Autodesk Inventor part; units mm, degrees
(part 2 of 2)
sketch "Magnet_flange_bottom_front" plane through (0, 0, -10) normal (0, 0, -1) x (-1, 0, 0)
  circle A0 centre (-365, 62.5) radius 1.65
  arc A1 (-385, 56.5) -> (-385, 68.5) centre (-385, 62.5) ccw
  line L0 (-355, 52.5) -> (-355, 72.5)
  line L1 (-355, 52.5) -> (-370, 52.5)
  circle A2 centre (-377.5, 45) radius 2.25
  line L2 (-370, 52.5) -> (-370, 37.5)
  line L3 (-385, 56.5) -> (-385, 37.5)
  line L4 (-385, 37.5) -> (-370, 37.5)
  line L5 (-385, 87.5) -> (-385, 68.5)
  line L6 (-370, 87.5) -> (-385, 87.5)
  line L7 (-370, 72.5) -> (-370, 87.5)
  line L8 (-355, 72.5) -> (-370, 72.5)
  circle A3 centre (-377.5, 80) radius 2.25
  point P0 (0, 0)
  dimension "d739" = 50
  dimension "d740" = 15
  dimension "d741" = 15
  dimension "d742" = 15
  dimension "d743" = 4.5
  dimension "d744" = 4.5
  dimension "d745" = 7.5
  dimension "d746" = 7.5
  dimension "d747" = 12
  dimension "d748" = 15
  dimension "d749" = 15
  dimension "d750" = 7.5
  dimension "d751" = 7.5
  dimension "d752" = 19
  dimension "d753" = 3.3
  dimension "d754" = 10
  dimension "d755" = 10
  constraints: 18 end point, 4 centre point, 3 parallel, 3 perpendicular, 2 line through centre, 2 point on circle, 1 coincident
  measures "d739" distance between parallel lines of L6 L4
  measures "d740" distance between parallel lines of L4 L1
  measures "d741" distance between parallel lines of L6 L8
  measures "d742" distance between parallel lines of L0 L2
  measures "d743" diameter of A2
  measures "d744" diameter of A3
  measures "d745" distance from line of L4 A2.centre
  measures "d746" distance from line of L6 A3.centre
  measures "d747" diameter of A1
  measures "d748" distance between parallel lines of L3 L2
  measures "d749" distance between parallel lines of L5 L7
  measures "d750" distance from line of L2 A2.centre
  measures "d751" distance from line of L7 A3.centre
  measures "d752" distance of L3.start L4.start
  measures "d753" diameter of A0
  measures "d754" distance from line of L1 A0.centre
  measures "d755" distance from line of L0 A0.centre
sketch "Magnet_flange_middle_front" plane through (0, 0, -10) normal (0, 0, -1) x (-1, 0, 0)
  circle A0 centre (-415, 355) radius 1.65
  arc A1 (-435, 349) -> (-435, 361) centre (-435, 355) ccw
  line L0 (-405, 345) -> (-405, 365)
  line L1 (-405, 345) -> (-420, 345)
  circle A2 centre (-427.5, 337.5) radius 2.25
  line L2 (-420, 345) -> (-420, 330)
  line L3 (-435, 349) -> (-435, 330)
  line L4 (-435, 330) -> (-420, 330)
  line L5 (-435, 380) -> (-435, 361)
  line L6 (-420, 380) -> (-435, 380)
  line L7 (-420, 365) -> (-420, 380)
  line L8 (-405, 365) -> (-420, 365)
  circle A3 centre (-427.5, 372.5) radius 2.25
  point P0 (0, 0)
  dimension "d756" = 50
  dimension "d757" = 15
  dimension "d758" = 15
  dimension "d759" = 15
  dimension "d760" = 4.5
  dimension "d761" = 4.5
  dimension "d762" = 7.5
  dimension "d763" = 7.5
  dimension "d764" = 12
  dimension "d765" = 15
  dimension "d766" = 15
  dimension "d767" = 7.5
  dimension "d768" = 7.5
  dimension "d769" = 19
  dimension "d770" = 3.3
  dimension "d771" = 10
  dimension "d772" = 10
  constraints: 18 end point, 4 centre point, 3 parallel, 3 perpendicular, 2 line through centre, 2 point on circle, 1 coincident
  measures "d756" distance between parallel lines of L6 L4
  measures "d757" distance between parallel lines of L4 L1
  measures "d758" distance between parallel lines of L6 L8
  measures "d759" distance between parallel lines of L0 L2
  measures "d760" diameter of A2
  measures "d761" diameter of A3
  measures "d762" distance from line of L4 A2.centre
  measures "d763" distance from line of L6 A3.centre
  measures "d764" diameter of A1
  measures "d765" distance between parallel lines of L3 L2
  measures "d766" distance between parallel lines of L5 L7
  measures "d767" distance from line of L2 A2.centre
  measures "d768" distance from line of L7 A3.centre
  measures "d769" distance of L3.start L3.end
  measures "d770" diameter of A0
  measures "d771" distance from line of L1 A0.centre
  measures "d772" distance from line of L0 A0.centre
extrude "Magnet_flange_middle_front_1" add sketch "Magnet_flange_middle_front" along normal blind 10 separate body
extrude "Magnet_flange_bottom_front_1" add sketch "Magnet_flange_bottom_front" along normal blind 10 separate body
sketch "Magnet_hole_top_door_front" plane through (0, 0, 10) normal (0, 0, 1) x (1, 0, 0)
  line L0 (185, 580) -> (375, 580) projected
  line L1 (380, 575) -> (380, 485) projected
  point P0 (0, 0)
  point P1 (390, 530)
  dimension "d811" = 50
  dimension "d812" = 10
  measures "d811" distance from line of point (390, 530) L0
  measures "d812" distance from line of L1 point (390, 530)
hole "Magnet_hole_top_door_front_1" at (390, 530, 10) direction (0, 0, -1) diameter 6.2 end through all bodies 1
sketch "Top_door_hinge_levellers_front_holes" plane through (0, 0, 10) normal (0, 0, 1) x (1, 0, 0)
  line L0 (565, 610) -> (0, 610) projected
  line L1 (0, 610) -> (0, 0) projected
  point P0 (147.3, 580.9)
  point P1 (147.3, 549.1)
  point P2 (147.3, 510.9)
  point P3 (147.3, 479.1)
  dimension "d850" = 29.1
  dimension "d851" = 147.3
  dimension "d852" = 31.8
  dimension "d853" = 147.3
  dimension "d854" = 99.1
  dimension "d855" = 147.3
  dimension "d856" = 31.8
  dimension "d857" = 147.3
  measures "d850" distance from line of L0 point (147.3, 580.9)
  measures "d851" distance from line of L1 point (147.3, 580.9)
  measures "d852" distance of point (147.3, 549.1) point (147.3, 580.9)
  measures "d853" distance from line of L1 point (147.3, 549.1)
  measures "d854" distance from line of L0 point (147.3, 510.9)
  measures "d855" distance from line of L1 point (147.3, 510.9)
  measures "d856" distance of point (147.3, 510.9) point (147.3, 479.1)
  measures "d857" distance from line of L1 point (147.3, 479.1)
hole "Top_door_hinge_leveller_front_holes" at (147.3, 580.9, 10) at (147.3, 549.1, 10) at (147.3, 510.9, 10) at (147.3, 479.1, 10) direction (0, 0, -1) diameter 3.3 end through all bodies 1
sketch "Window_holes" plane through (0, 0, -10) normal (0, 0, -1) x (-1, 0, 0)
  line L0 (-165, 585) -> (-395, 585) projected
  line L1 (-395, 475) -> (-165, 475) projected
  line L2 (-165, 475) -> (-165, 585) projected
  line L3 (-395, 585) -> (-395, 535) projected
  line L4 (-395, 525) -> (-395, 475) projected
  point P0 (0, 0)
  point P1 (-387.5, 565)
  point P2 (-387.5, 495)
  point P3 (-172.5, 495)
  point P4 (-172.5, 565)
  dimension "d1016" = 20
  dimension "d1017" = 20
  dimension "d1018" = 20
  dimension "d1019" = 20
  dimension "d1020" = 7.5
  dimension "d1021" = 7.5
  dimension "d1022" = 7.5
  dimension "d1023" = 7.5
  measures "d1016" distance from line of L0 point (-387.5, 565)
  measures "d1017" distance from line of L1 point (-387.5, 495)
  measures "d1018" distance from line of L1 point (-172.5, 495)
  measures "d1019" distance from line of L0 point (-172.5, 565)
  measures "d1020" distance from line of L2 point (-172.5, 565)
  measures "d1021" distance from line of L2 point (-172.5, 495)
  measures "d1022" distance from line of L3 point (-387.5, 565)
  measures "d1023" distance from line of L4 point (-387.5, 495)
hole "Window_holes_front" at (387.5, 565, -10) at (172.5, 565, -10) at (172.5, 495, -10) at (387.5, 495, -10) direction (0, 0, 1) diameter 4.5 end through all bodies 6 clearance for "Countersunk Flat Head Screw DIN EN ISO 2009" size "M4" standard "DIN"
